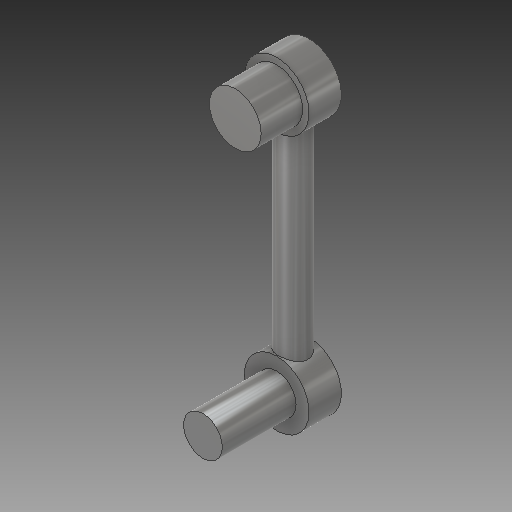
# Autodesk Inventor part: 101-03
Saved by Autodesk Inventor 2019 (Build 230136000, 136)
## iProperties
Company: Autodesk Inc.
Created: 2017-03-15
Part Number: 101-03
Material: Aluminum 6061
Document SubType Name: Modeling
Designer: Autodesk Inc.
Density: 2.7 g/cm^3
Appearance: Aluminum - Anodized Glossy (Grey)
Mass: 0.58869 g
Surface Area: 3.77539 cm^2
Volume: 0.218033 cm^3
Author: Inventor
Autodesk Inventor part; units mm, degrees
ref_plane "YZ Plane" through (0, 0, 0) normal (1, 0, 0) x (0, 1, 0)
ref_plane "XZ Plane" through (0, 0, 0) normal (0, 1, 0) x (-1, 0, 0)
ref_plane "XY Plane" through (0, 0, 0) normal (0, 0, 1) x (1, 0, 0)
sketch "Sketch1" plane through (0, 0, 0) normal (0, 1, 0) x (-1, 0, 0)
  circle A0 centre (0, 0) radius 1.15
  dimension "d0" = 2.3
  constraints: 1 centre point, 1 coincident
  measures "d0" diameter of A0
extrude "Extrusion1" add sketch "Sketch1" along normal blind 16
sketch "Sketch2" plane through (0, 0, 0) normal (1, 0, 0) x (0, 1, 0)
  line L0 (16, -1.15) -> (16, 1.15) projected
  line L1 (15.5, 1.25) -> (15.5, 0)
  line L2 (16, 0) -> (15.5, 0)
  line L3 (15.5, 0) -> (13.7557, 0)
  line L4 (15.5, 1.25) -> (18, 1.25)
  line L5 (18, 1.25) -> (18, 0)
  line L6 (16, 1.15) -> (16, -1.15)
  line L7 (15.5, -1.25) -> (15.5, 0)
  line L8 (15.5, -1.25) -> (18, -1.25)
  line L9 (18, -1.25) -> (18, 0)
  point P0 (0, 0)
  dimension "d3" = 0.5
  dimension "d4" = 1.25
  dimension "d7" = 2.5
  constraints: 18 end point, 4 symmetric about line, 2 horizontal, 2 vertical, 1 midpoint, 1 perpendicular, 1 point on line
  measures "d3" distance between parallel lines of L1 L0
  measures "d4" distance of L1.end L1.start
  measures "d7" distance between parallel lines of L5 L1
revolve "Revolution1" add sketch "Sketch2" angle 360 about axis through (0, 18, 1.25) along (0, 0, -1)
sketch "Sketch3" plane through (0, 18, 1.25) normal (0, 0, 1) x (1, 0, 0)
  circle A0 centre (0, 0) radius 2.5 projected
  circle A1 centre (0, 0) radius 2
  point P0 (0, -18)
  dimension "d9" = 4
  constraints: 1 centre point, 1 coincident
  measures "d9" diameter of A1
extrude "Extrusion2" add sketch "Sketch3" along normal blind 3.2 contours A1
sketch "Sketch4" plane through (0, 18, -1.25) normal (0, 0, -1) x (-1, 0, 0)
  circle A0 centre (0, 0) radius 2 projected
  point P0 (0, -18)
extrude "Extrusion3" cut sketch "Sketch4" against normal blind 1.6
sketch "Sketch5" plane through (0, 0, 0) normal (1, 0, 0) x (0, 1, 0)
  line L0 (0.5, 0) -> (0.5, -1.25)
  line L1 (0, 1.15) -> (0, -1.15) projected
  line L2 (0, 0) -> (0.5, 0)
  line L3 (0.5, 0) -> (1.4582, 0)
  line L4 (0.5, 0) -> (0.5, -1.25)
  line L5 (-2, 0) -> (-2, -1.25)
  line L6 (0.5, -1.25) -> (-2, -1.25)
  line L7 (0.5, 0) -> (0.5, 1.25)
  line L8 (0, -1.15) -> (0, 1.15)
  line L9 (0.5, 0) -> (0.5, 1.25)
  line L10 (-2, 0) -> (-2, 1.25)
  line L11 (0.5, 1.25) -> (-2, 1.25)
  dimension "d14" = 0.5
  dimension "d15" = 1.25
  dimension "d16" = 2.5
  constraints: 22 end point, 4 symmetric about line, 2 horizontal, 2 vertical, 1 perpendicular, 1 point on line
  measures "d14" distance between parallel lines of L1 L0
  measures "d15" distance of L0.start L0.end
  measures "d16" distance between parallel lines of L5 L0
revolve "Revolution2" add sketch "Sketch5" angle 360 about axis through (0, -2, 0) along (0, 0, 1)
sketch "Sketch6" plane through (0, -2, 1.25) normal (0, 0, 1) x (1, 0, 0)
  circle A0 centre (0, 0) radius 2.5 projected
  circle A1 centre (0, 0) radius 1.5
  point P0 (0, 2)
  dimension "d18" = 3
  constraints: 1 centre point, 1 coincident
  measures "d18" diameter of A1
extrude "Extrusion4" add sketch "Sketch6" along normal blind 5.7 contours A1
sketch "Sketch7" plane through (0, -2, -1.25) normal (0, 0, -1) x (-1, 0, 0)
  circle A0 centre (0, 0) radius 1.5 projected
  point P0 (0, 2)
extrude "Extrusion5" cut sketch "Sketch7" against normal blind 0.5
body "Solid1"
